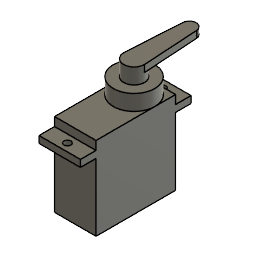
ServoMotor (Autodesk Fusion 360 design; units mm, degrees)
part number: 2025-11-07-13-28-11-303
Autodesk Fusion 360 part; units mm, degrees
sketch "Boceto1" plane through (0, 0, 0) normal (0, 1, 0) x (1, 0, 0)
  line L0 (-25, 25) -> (-25, 2)
  line L1 (-25, 25) -> (-13, 25)
  line L2 (-13, 25) -> (-13, 2)
  line L3 (-25, 2) -> (-13, 2)
  dimension "d1" = 23
  dimension "d2" = 12
  constraint vertical L0
  constraint perpendicular L0 L1
  constraint perpendicular L1 L2
  constraint perpendicular L2 L3
  measures "d1" distance of L0.start L0.end
  measures "d2" distance of L0.start L1.end
extrude "Extruir1" add sketch "Boceto1" along normal blind 24
sketch "Boceto2" plane through (0, 0, -2) normal (0, 0, 1) x (1, 0, 0)
  line L0 (-25, 0) -> (-13, 0)
  line L1 (-13, 0) -> (-13, 24)
  line L2 (-13, 24) -> (-25, 24)
  line L3 (-25, 24) -> (-25, 0)
  line L4 (-13, 19.5) -> (-25, 19.5)
  line L5 (-25, 19.5) -> (-25, 21.5)
  line L6 (-25, 21.5) -> (-13, 21.5)
  line L7 (-13, 21.5) -> (-13, 19.5)
  dimension "d5" = 19.5
  dimension "d6" = 2
  constraint coincident L3 L4.end
  constraint perpendicular L3 L4
  constraint perpendicular L2 L5
  constraint coincident L1 L6.end
  constraint perpendicular L1 L6
  measures "d5" distance of L0.end L4.start
  measures "d6" distance of L4.end L5.end
extrude "Extruir2" add sketch "Boceto2" along normal blind 4.5 contours L1 L3 L4 L5 L6 L7
sketch "Boceto3" plane through (0, 0, -25) normal (0, 0, -1) x (-1, 0, 0)
  line L0 (13, 0) -> (25, 0)
  line L1 (25, 0) -> (25, 24)
  line L2 (25, 24) -> (13, 24)
  line L3 (13, 24) -> (13, 0)
  line L4 (25, 19.5) -> (13, 19.5)
  line L5 (13, 19.5) -> (13, 21.5)
  line L6 (13, 21.5) -> (25, 21.5)
  line L7 (25, 21.5) -> (25, 19.5)
  dimension "d9" = 19.5
  dimension "d10" = 2
  constraint coincident L3 L4.end
  constraint perpendicular L3 L4
  constraint perpendicular L4 L5
  constraint coincident L1 L6.end
  constraint perpendicular L1 L6
  measures "d9" distance of L0.end L4.start
  measures "d10" distance of L4.end L5.end
extrude "Extruir3" add sketch "Boceto3" along normal blind 4.5 contours L1 L3 L4 L5 L6 L7
sketch "Boceto4" plane through (0, 21.5, 0) normal (0, 1, 0) x (-1, 0, 0)
  line L0 (13, -2) -> (25, -2)
  line L1 (25, -2) -> (25, 2.5)
  line L2 (25, 2.5) -> (13, 2.5)
  line L3 (13, 2.5) -> (13, -2)
  circle A0 centre (19, 0.25) radius 1
  dimension "d13" = 2
  measures "d13" diameter of A0
sketch "Boceto5" plane through (0, 21.5, 0) normal (0, 1, 0) x (-1, 0, 0)
  line L0 (25, -25) -> (13, -25)
  line L1 (13, -25) -> (13, -29.5)
  line L2 (13, -29.5) -> (25, -29.5)
  line L3 (25, -29.5) -> (25, -25)
  circle A0 centre (19, -27.25) radius 1
  dimension "d14" = 2
  measures "d14" diameter of A0
extrude "Extruir4" cut sketch "Boceto4" sketch "Boceto5" against normal blind 5 contours A0 of sketch 2 contours A0
sketch "Boceto6" plane through (0, 24, 0) normal (0, 1, 0) x (-1, 0, 0)
  line L0 (25, -25) -> (25, -2)
  line L1 (25, -2) -> (13, -2)
  line L2 (13, -2) -> (13, -25)
  line L3 (13, -25) -> (25, -25)
  line L4 (13, -25) -> (13, -19)
  circle A0 centre (19, -19) radius 6
  constraint coincident L2.end L3.start
  constraint coincident L2 L4.end
  constraint tangent L0 A0
extrude "Extruir5" add sketch "Boceto6" along normal blind 4.5 contours A0
sketch "Boceto7" plane through (0, 28.5, 0) normal (0, 1, 0) x (-1, 0, 0)
  circle A0 centre (19, -19) radius 6
  circle A1 centre (19, -19) radius 3
  dimension "d19" = 6
  constraint concentric A0 A1
  measures "d19" diameter of A1
extrude "Extruir6" add sketch "Boceto7" along normal blind 2.5 contours A1
sketch "Boceto8" plane through (0, 31, 0) normal (0, 1, 0) x (-1, 0, 0)
  line L0 (22, -19) -> (20.995, -35.1418)
  line L1 (16, -19) -> (17.005, -35.1418)
  arc A0 (22, -19) -> (16, -19) centre (19, -19) ccw
  arc A1 (17.005, -35.1418) -> (20.995, -35.1418) centre (19, -35) ccw
extrude "Extruir7" add sketch "Boceto8" along normal blind 2
